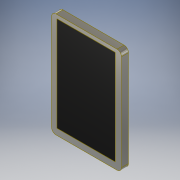
# Autodesk Inventor part: Logo
Saved by Autodesk Inventor 2018 (Build 220112000, 112)
## iProperties
Created: 2019-02-22
Part Number: Logo
Material: Generic
Document SubType Name: Modeling
Designer: This kid
Density: 1 g/cm^3
Appearance: Silver
Author: This kid
Autodesk Inventor part; units mm, degrees
ref_plane "YZ Plane" through (0, 0, 0) normal (1, 0, 0) x (0, 1, 0)
ref_plane "XZ Plane" through (0, 0, 0) normal (0, 1, 0) x (-1, 0, 0)
ref_plane "XY Plane" through (0, 0, 0) normal (0, 0, 1) x (1, 0, 0)
sketch "Sketch1" plane through (0, 0, 0) normal (0, 0, 1) x (1, 0, 0)
  line L0 (-22.225, -38.1) -> (22.225, -38.1)
  line L1 (25.4, -34.925) -> (25.4, 34.925)
  line L2 (22.225, 38.1) -> (-22.225, 38.1)
  line L3 (-25.4, 34.925) -> (-25.4, -34.925)
  line L4 (-25.4, -38.1) -> (25.4, 38.1) construction
  line L5 (25.4, -38.1) -> (-25.4, 38.1) construction
  arc A0 (-22.225, 38.1) -> (-25.4, 34.925) centre (-22.225, 34.925) ccw
  arc A1 (25.4, 34.925) -> (22.225, 38.1) centre (22.225, 34.925) ccw
  arc A2 (22.225, -38.1) -> (25.4, -34.925) centre (22.225, -34.925) ccw
  arc A3 (-25.4, -34.925) -> (-22.225, -38.1) centre (-22.225, -34.925) ccw
  point P0 (0, 0)
  dimension "d0" = 50.8
  dimension "d1" = 76.2
  dimension "d2" = 3.175
  constraints: 12 end point, 8 point on circle, 8 point on line, 8 tangent, 4 centre point, 3 equal radius, 2 midpoint, 2 parallel, 1 horizontal, 1 perpendicular
  measures "d0" distance of L5.end L4.end
  measures "d1" distance of L4.end L5.start
  measures "d2" radius of A0
extrude "Extrusion1" add sketch "Sketch1" along normal blind 5.08
sketch "Sketch2" plane through (0, 0, 5.08) normal (0, 0, 1) x (1, 0, 0)
  line L0 (-21.5129, 35.362) -> (20.875, 35.362)
  line L1 (20.875, 35.362) -> (20.875, -33.5369)
  line L2 (20.875, -33.5369) -> (-21.5129, -33.5369)
  line L3 (-21.5129, -33.5369) -> (-21.5129, 35.362)
  point P0 (0, 0)
  constraints: 8 end point, 3 perpendicular, 1 horizontal
extrude "Extrusion2" add sketch "Sketch2" along normal blind 0.0254
body "Solid1"
